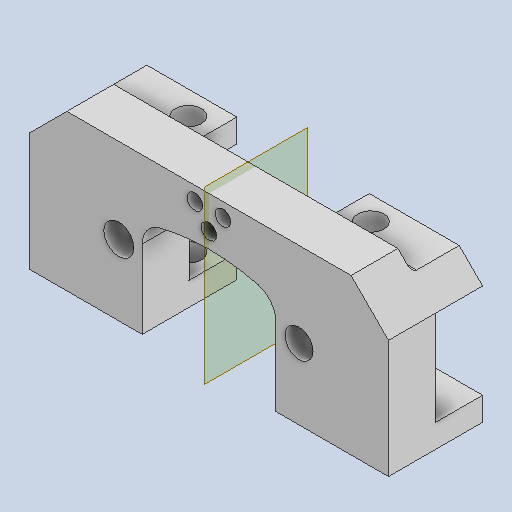
# Autodesk Inventor part: pivot module base
Saved by Autodesk Inventor 2022 (Build 260153000, 153)
## iProperties
Created: 2021-12-08
Part Number: pivot module base
Material: Generic
Document SubType Name: Modeling
Designer: efred
Density: 1 g/cm^3
Appearance: Default
Author: efred
Autodesk Inventor part; units mm, degrees
ref_plane "YZ Plane" through (0, 0, 0) normal (1, 0, 0) x (0, 1, 0)
sketch "Sketch1" plane through (0, 0, 0) normal (0, 0, 1) x (1, 0, 0)
  circle A0 centre (0, 0) radius 3.1 construction
  line L0 (-5, 10) -> (-5, -10) projected
  line L1 (-5, -10) -> (19.1, -10) construction
  line L2 (19.1, -10) -> (19.1, 10) projected
  line L3 (19.1, 10) -> (-5, 10) construction
  line L4 (-33.5, -10) -> (-33.5, 10) projected
  line L5 (-33.5, 10) -> (-57.6, 10) construction
  line L6 (-57.6, -10) -> (-57.6, 10) projected
  line L7 (-57.6, -10) -> (-33.5, -10) construction
  circle A1 centre (-38.5, 0) radius 3.1 construction
  line L8 (-25.05, 5.3172) -> (-13.45, 5.3172) projected
  line L9 (19.1, -10.1) -> (-5, -10.1)
  line L10 (-5, -10.1) -> (-5, 1.6198)
  line L11 (-5, 10.1) -> (19.1, 10.1)
  line L12 (19.1, 10.1) -> (19.1, -10.1)
  line L13 (-33.5, -10.1) -> (-57.6, -10.1)
  line L14 (-57.6, -10.1) -> (-57.6, 10.1)
  line L15 (-57.6, 10.1) -> (-33.5, 10.1)
  line L16 (-33.5, 1.6198) -> (-33.5, -10.1)
  circle A2 centre (-38.5, 0) radius 3.2
  circle A3 centre (0, 0) radius 3
  arc A4 (-8.7654, 6.465) -> (-29.7346, 6.465) centre (-19.25, -34.6828) ccw
  line L17 (11.1, 18.1) -> (-49.6, 18.1)
  line L18 (-19.25, 5.3172) -> (-19.25, 9.0349) construction
  circle A5 centre (-16.25, 15.1) radius 1.65
  circle A6 centre (-22.25, 15.1) radius 1.65
  line L19 (11.1, 18.1) -> (19.1, 10.1)
  line L20 (-49.6, 18.1) -> (-57.6, 10.1)
  arc A7 (-29.7346, 6.465) -> (-33.5, 1.6198) centre (-28.5, 1.6198) ccw
  arc A8 (-5, 1.6198) -> (-8.7654, 6.465) centre (-10, 1.6198) ccw
  circle A9 centre (-19.25, 11.1) radius 1.65
  circle A10 centre (-19.25, 11.1) radius 1.65
  point P0 (0, 0)
  point P1 (-5, 5.3172)
  point P2 (-33.5, 5.3172)
  point P3 (-19.25, 18.1)
  point P4 (-5, 5.3172)
  point P5 (19.1, 10)
  point P6 (-33.5, 1.6198)
  point P7 (-5, 1.6198)
  dimension "d0" = 0.1
  dimension "d1" = 0.1
  dimension "d2" = 0.1
  dimension "d3" = 0.1
  dimension "d4" = 0.1
  dimension "d5" = 0.1
  dimension "d7" = 40
  dimension "d9" = 8
  dimension "d10" = 3
  dimension "d11" = 3.3
  dimension "d12" = 3
  dimension "d13" = 45
  dimension "d16" = 5
  dimension "d17" = 3.3
  dimension "d19" = 7
  constraints: 24 end point, 9 centre point, 8 point on circle, 5 point on line, 4 collinear, 4 parallel, 4 tangent, 3 horizontal, 3 horizontal alignment, 2 equal radius, 2 midpoint, 2 perpendicular, 2 vertical alignment, 1 coincident, 1 vertical, 1 other
  measures "d0" distance between parallel lines of L1 L9
  measures "d1" distance between parallel lines of L3 L11
  measures "d2" distance between parallel lines of L5 L15
  measures "d3" distance between parallel lines of L7 L13
  measures "d4" radial gap between concentric circles of A1 A2
  measures "d5" radial gap between concentric circles of A0 A3
  measures "d7" distance from line of L8 A4.centre
  measures "d9" distance between parallel lines of L11 L17
  measures "d10" distance from line of L18 A5.centre
  measures "d11" diameter of A5
  measures "d12" distance from line of L17 A5.centre
  measures "d13" angle of L11 L19
  measures "d16" radius of A7
  measures "d17" diameter of A9
  measures "d19" distance of point (-19.25, 18.1) A9.centre
extrude "Extrusion1" add sketch "Sketch1" along normal blind 10
ref_plane "Work Plane1" through (-43.1, -10, -10.1) normal (0, 0, -1) x (0, 1, 0)
sketch "Sketch3" plane through (0, 0, 10) normal (0, 0, 1) x (1, 0, 0)
  line L0 (-33.5, -10.1) -> (-33.5, 1.6198) projected
  line L1 (-33.5, -10.1) -> (-57.6, -10.1)
  line L2 (-57.6, -10.1) -> (-57.6, -15.1)
  line L3 (-57.6, -15.1) -> (-33.5, -15.1)
  line L4 (-33.5, -15.1) -> (-33.5, -10.1)
  line L5 (-57.6, 10.1) -> (-57.6, -10.1) projected
  point P0 (0, 0)
  dimension "d25" = 5
  constraints: 8 end point, 2 parallel, 1 collinear, 1 horizontal, 1 perpendicular
  measures "d25" distance between parallel lines of L1 L3
extrude "Extrusion3" add sketch "Sketch3" against normal up to surface (20.1 mm away)
sketch "Sketch4" plane through (0, 0, 0) normal (0, 0, -1) x (-1, 0, 0)
  line L0 (33.5, -10) -> (33.5, 10) construction
  line L1 (33.5, 10) -> (57.6, 10) construction
  line L2 (57.6, -10) -> (57.6, 10) construction
  line L3 (57.6, -10) -> (33.5, -10) construction
  circle A0 centre (38.5, 0) radius 3.1 construction
  line L4 (-19.1, -10.1) -> (-19.1, 10.1) construction
  line L5 (5, -10.1) -> (-19.1, -10.1) construction
  line L6 (5, 1.6198) -> (5, -10.1) construction
  arc A1 (8.7654, 6.465) -> (5, 1.6198) centre (10, 1.6198) ccw construction
  arc A2 (29.7346, 6.465) -> (8.7654, 6.465) centre (19.25, -34.6828) ccw construction
  arc A3 (33.5, 1.6198) -> (29.7346, 6.465) centre (28.5, 1.6198) ccw construction
  line L7 (33.5, -10.1) -> (33.5, 1.6198) construction
  line L8 (57.6, -10.1) -> (33.5, -10.1) construction
  line L9 (57.6, 10.1) -> (57.6, -10.1) construction
  line L10 (49.6, 18.1) -> (57.6, 10.1) projected
  line L11 (-11.1, 18.1) -> (49.6, 18.1) construction
  line L12 (-19.1, 10.1) -> (-11.1, 18.1) construction
  circle A4 centre (19.25, 11.1) radius 1.65 construction
  circle A5 centre (16.25, 15.1) radius 1.65 construction
  circle A6 centre (0, 0) radius 3 construction
  circle A7 centre (38.5, 0) radius 3.2 construction
  circle A8 centre (22.25, 15.1) radius 1.65 construction
  line L13 (57.7, 10.1) -> (33.4, 10.1)
  line L14 (33.4, 10.1) -> (33.4, -10.1) construction
  line L15 (33.4, -10.1) -> (57.7, -10.1) construction
  line L16 (57.7, -10.1) -> (57.7, 10.1) construction
  line L17 (33.4, 10.1) -> (33.4, 18.1)
  line L18 (-11.1, 18.1) -> (49.6, 18.1) projected
  line L19 (49.6, 18.1) -> (57.6, 10.1) projected
  line L20 (33.4, 18.1) -> (49.6, 18.1)
  point P0 (0, 0)
  dimension "d28" = 0.1
  constraints: 12 end point, 2 perpendicular, 1 point on line, 3 other
  measures "d28" distance between parallel lines of L1 L13
ref_plane "Work Plane2" through (-43.1, -10, -10.1) normal (0, 0, -1) x (0, 1, 0)
extrude "Extrusion4" add sketch "Sketch4" along normal up to surface (10.1 mm away)
sketch "Sketch5" plane through (-49.6, 18.1, 10) normal (0, 1, 0) x (1, 0, 0)
  line L0 (16.1, 20.1) -> (16.1, 10.1) construction
  line L1 (-8, 10.1) -> (16.1, 10.1) construction
  line L2 (-8, 302.9) -> (-8, 10.1) construction
  line L3 (-8, 302.9) -> (68.7, 302.9) construction
  line L4 (68.7, 10.1) -> (68.7, 302.9) construction
  line L5 (44.6, 10.1) -> (68.7, 10.1) construction
  line L6 (44.6, 10.1) -> (44.6, 20.1) construction
  line L7 (44.6, 20.1) -> (54.2, 20.1) construction
  arc A0 (54.2, 20.1) -> (59.2, 25.1) centre (54.2, 25.1) ccw construction
  line L8 (59.2, 175.1) -> (59.2, 25.1) construction
  arc A1 (59.2, 175.1) -> (54.2, 180.1) centre (54.2, 175.1) ccw construction
  line L9 (6.5, 180.1) -> (54.2, 180.1) construction
  arc A2 (6.5, 180.1) -> (1.5, 175.1) centre (6.5, 175.1) ccw construction
  line L10 (1.5, 25.1) -> (1.5, 175.1) construction
  arc A3 (1.5, 25.1) -> (6.5, 20.1) centre (6.5, 25.1) ccw construction
  line L11 (16.1, 20.1) -> (6.5, 20.1) construction
  circle A4 centre (63.7, 292.9) radius 2.15 construction
  circle A5 centre (-3, 273) radius 2.15 construction
  circle A6 centre (-3, 292.9) radius 2.15 construction
  circle A7 centre (63.7, 273) radius 2.15 construction
  circle A8 centre (10.85, 15.1) radius 2.5 construction
  circle A9 centre (49.85, 15.1) radius 2.5 construction
  line L12 (-8, 10) -> (-8, 20.1) projected
  line L13 (16.2, 10) -> (16.2, 20.1) projected
  line L14 (-8, 10) -> (16.2, 10)
  line L15 (16.2, 10) -> (16.2, 20.1)
  line L16 (16.2, 20.1) -> (-8, 20.1)
  line L17 (-8, 20.1) -> (-8, 10)
  point P0 (49.6, 10)
  constraints: 8 end point, 2 parallel, 1 horizontal, 1 perpendicular
extrude "Extrusion5" cut sketch "Sketch5" against normal blind 3
sketch "Sketch6" plane through (-49.6, 15.1, 10) normal (0, 1, 0) x (1, 0, 0)
  circle A0 centre (10.85, 15.1) radius 2.5 construction
  circle A1 centre (10.85, 15.1) radius 2.8
  point P0 (49.6, 10)
  dimension "d33" = 0.3
  constraints: 1 centre point
  measures "d33" radial gap between concentric circles of A0 A1
extrude "Extrusion6" cut sketch "Sketch6" against normal through all
fillet "Fillet2" radius 1 1 edges at (-43, 15.1, 0)
ref_plane "Work Plane3" through (-19.25, -15.1, 10) normal (-1, 0, 0) x (0, 0, 1)
mirror "Mirror1" about plane through (-19.25, -15.1, 10) normal (-1, 0, 0) of "Extrusion3", "Extrusion4", "Extrusion5", "Extrusion6", "Fillet2"
ref_plane "Work Plane4" through (4.6, -10, -10.1) normal (0, 0, 1) x (0, 1, 0)
equation "\"d17\" = d11"
body "Solid1"
